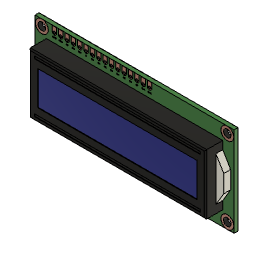
Control Panel v4 (Autodesk Fusion 360 archive; units mm, degrees)
design "LCD screen"
Autodesk Fusion 360 part; units mm, degrees
(part 1 of 2)
sketch "Boceto1" plane through (0, 0, 0) normal (0, 1, 0) x (1, 0, 0)
  line L0 (40.08, -18.04) -> (-40.08, -18.04)
  line L1 (-40.08, -18.04) -> (-40.08, 18.04)
  line L2 (-40.08, 18.04) -> (40.08, 18.04)
  line L3 (40.08, 18.04) -> (40.08, -18.04)
  line L4 (40.08, -18.04) -> (-40.08, 18.04) construction
  line L5 (-40.08, -18.04) -> (40.08, 18.04) construction
  dimension "d1" = 80.16
  dimension "d2" = 36.08
  constraint horizontal L0
  constraint perpendicular L0 L1
  constraint parallel L0 L2
  constraint parallel L1 L3
  constraint coincident L4 origin
  constraint coincident L5 origin
  measures "d1" distance of L0.start L0.end
  measures "d2" distance of L0.start L2.end
extrude "Extruir1" add sketch "Boceto1" along normal blind 1.61
sketch "Boceto2" plane through (0, 0, 0) normal (0, -1, 0) x (1, 0, 0)
  line L0 (-40.08, -18.04) -> (40.08, -18.04)
  line L1 (40.08, -18.04) -> (40.08, 18.04)
  line L2 (40.08, 18.04) -> (-40.08, 18.04)
  line L3 (-40.08, 18.04) -> (-40.08, -18.04)
  line L4 (0, 0) -> (0, 18.04) construction
  line L5 (0, 0) -> (40.08, 0) construction
  circle A0 centre (37.355, 15.465) radius 1.525
  circle A1 centre (37.355, 15.465) radius 2.595
  circle A2 centre (-37.355, 15.465) radius 1.525
  circle A3 centre (-37.355, 15.465) radius 2.595
  circle A4 centre (-37.355, -15.465) radius 1.525
  circle A5 centre (-37.355, -15.465) radius 2.595
  circle A6 centre (37.355, -15.465) radius 1.525
  circle A7 centre (37.355, -15.465) radius 2.595
  line L6 (35.525, 12.1) -> (-35.525, 12.1)
  line L7 (-35.525, 12.1) -> (-35.525, -12.1)
  line L8 (-35.525, -12.1) -> (35.525, -12.1)
  line L9 (35.525, -12.1) -> (35.525, 12.1)
  line L10 (35.525, 12.1) -> (-35.525, -12.1) construction
  line L11 (-35.525, 12.1) -> (35.525, -12.1) construction
  line L12 (35.525, 8.88) -> (38.695, 8.88)
  line L13 (38.695, 8.88) -> (38.695, -8.88)
  line L14 (38.695, -8.88) -> (35.525, -8.88)
  line L15 (35.525, -8.88) -> (35.525, 8.88)
  line L16 (38.695, 3.54) -> (35.525, 8.88)
  line L17 (38.695, -3.54) -> (35.525, -8.88)
  line L18 (-33.18, 17.94) -> (-31.43, 17.94)
  line L19 (-31.43, 17.94) -> (-31.43, 15.815)
  line L20 (-33.18, 15.815) -> (-33.18, 17.94)
  line L21 (-31.43, 17.94) -> (-33.18, 15.815) construction
  line L22 (-31.43, 15.815) -> (-33.18, 17.94) construction
  line L23 (-32.305, 14.94) -> (-33.18, 14.94) construction
  line L24 (-33.18, 15.815) -> (-33.18, 14.94) construction
  arc A8 (-33.18, 15.815) -> (-31.43, 15.815) centre (-32.305, 15.815) ccw
  line L25 (-32.305, 16.8775) -> (-32.305, 14.94) construction
  line L26 (-30.6233, 17.94) -> (-28.8733, 17.94)
  line L27 (-30.6233, 15.815) -> (-30.6233, 17.94)
  arc A9 (-30.6233, 15.815) -> (-28.8733, 15.815) centre (-29.7483, 15.815) ccw
  line L28 (-28.8733, 17.94) -> (-28.8733, 15.815)
  line L29 (-28.0667, 17.94) -> (-26.3167, 17.94)
  line L30 (-28.0667, 15.815) -> (-28.0667, 17.94)
  arc A10 (-28.0667, 15.815) -> (-26.3167, 15.815) centre (-27.1917, 15.815) ccw
  line L31 (-26.3167, 17.94) -> (-26.3167, 15.815)
  line L32 (-25.51, 17.94) -> (-23.76, 17.94)
  line L33 (-25.51, 15.815) -> (-25.51, 17.94)
  arc A11 (-25.51, 15.815) -> (-23.76, 15.815) centre (-24.635, 15.815) ccw
  line L34 (-23.76, 17.94) -> (-23.76, 15.815)
  line L35 (-22.9533, 17.94) -> (-21.2033, 17.94)
  line L36 (-22.9533, 15.815) -> (-22.9533, 17.94)
  arc A12 (-22.9533, 15.815) -> (-21.2033, 15.815) centre (-22.0783, 15.815) ccw
  line L37 (-21.2033, 17.94) -> (-21.2033, 15.815)
  line L38 (-20.3967, 17.94) -> (-18.6467, 17.94)
  line L39 (-20.3967, 15.815) -> (-20.3967, 17.94)
  arc A13 (-20.3967, 15.815) -> (-18.6467, 15.815) centre (-19.5217, 15.815) ccw
  line L40 (-18.6467, 17.94) -> (-18.6467, 15.815)
  line L41 (-17.84, 17.94) -> (-16.09, 17.94)
  line L42 (-17.84, 15.815) -> (-17.84, 17.94)
  arc A14 (-17.84, 15.815) -> (-16.09, 15.815) centre (-16.965, 15.815) ccw
  line L43 (-16.09, 17.94) -> (-16.09, 15.815)
  line L44 (-15.2833, 17.94) -> (-13.5333, 17.94)
  line L45 (-15.2833, 15.815) -> (-15.2833, 17.94)
  arc A15 (-15.2833, 15.815) -> (-13.5333, 15.815) centre (-14.4083, 15.815) ccw
  line L46 (-13.5333, 17.94) -> (-13.5333, 15.815)
  line L47 (-12.7267, 17.94) -> (-10.9767, 17.94)
  line L48 (-12.7267, 15.815) -> (-12.7267, 17.94)
  arc A16 (-12.7267, 15.815) -> (-10.9767, 15.815) centre (-11.8517, 15.815) ccw
  line L49 (-10.9767, 17.94) -> (-10.9767, 15.815)
  line L50 (-10.17, 17.94) -> (-8.42, 17.94)
  line L51 (-10.17, 15.815) -> (-10.17, 17.94)
  arc A17 (-10.17, 15.815) -> (-8.42, 15.815) centre (-9.295, 15.815) ccw
  line L52 (-8.42, 17.94) -> (-8.42, 15.815)
  line L53 (-7.6133, 17.94) -> (-5.8633, 17.94)
  line L54 (-7.6133, 15.815) -> (-7.6133, 17.94)
  arc A18 (-7.6133, 15.815) -> (-5.8633, 15.815) centre (-6.7383, 15.815) ccw
  line L55 (-5.8633, 17.94) -> (-5.8633, 15.815)
  line L56 (-5.0567, 17.94) -> (-3.3067, 17.94)
  line L57 (-5.0567, 15.815) -> (-5.0567, 17.94)
  arc A19 (-5.0567, 15.815) -> (-3.3067, 15.815) centre (-4.1817, 15.815) ccw
  line L58 (-3.3067, 17.94) -> (-3.3067, 15.815)
  line L59 (-2.5, 17.94) -> (-0.75, 17.94)
  line L60 (-2.5, 15.815) -> (-2.5, 17.94)
  arc A20 (-2.5, 15.815) -> (-0.75, 15.815) centre (-1.625, 15.815) ccw
  line L61 (-0.75, 17.94) -> (-0.75, 15.815)
  line L62 (0.0567, 17.94) -> (1.8067, 17.94)
  line L63 (0.0567, 15.815) -> (0.0567, 17.94)
  arc A21 (0.0567, 15.815) -> (1.8067, 15.815) centre (0.9317, 15.815) ccw
  line L64 (1.8067, 17.94) -> (1.8067, 15.815)
  line L65 (2.6133, 17.94) -> (4.3633, 17.94)
  line L66 (2.6133, 15.815) -> (2.6133, 17.94)
  arc A22 (2.6133, 15.815) -> (4.3633, 15.815) centre (3.4883, 15.815) ccw
  line L67 (4.3633, 17.94) -> (4.3633, 15.815)
  line L68 (5.17, 17.94) -> (6.92, 17.94)
  line L69 (5.17, 15.815) -> (5.17, 17.94)
  arc A23 (5.17, 15.815) -> (6.92, 15.815) centre (6.045, 15.815) ccw
  line L70 (6.92, 17.94) -> (6.92, 15.815)
  circle A24 centre (-32.305, 15.815) radius 0.5
  circle A25 centre (-29.7483, 15.815) radius 0.5
  circle A26 centre (-27.1917, 15.815) radius 0.5
  circle A27 centre (-24.635, 15.815) radius 0.5
  circle A28 centre (-22.0783, 15.815) radius 0.5
  circle A29 centre (-19.5217, 15.815) radius 0.5
  circle A30 centre (-16.965, 15.815) radius 0.5
  circle A31 centre (-14.4083, 15.815) radius 0.5
  circle A32 centre (-11.8517, 15.815) radius 0.5
  circle A33 centre (-9.295, 15.815) radius 0.5
  circle A34 centre (-6.7383, 15.815) radius 0.5
  circle A35 centre (-4.1817, 15.815) radius 0.5
  circle A36 centre (-1.625, 15.815) radius 0.5
  circle A37 centre (0.9317, 15.815) radius 0.5
  circle A38 centre (3.4883, 15.815) radius 0.5
  circle A39 centre (6.045, 15.815) radius 0.5
  line L71 (-32.305, 14.94) -> (-32.305, 12.1) construction
  line L72 (-33.18, 14.5) -> (-31.43, 14.5)
  line L73 (-31.43, 14.5) -> (-31.43, 13.6)
  line L74 (-31.43, 13.6) -> (-33.18, 13.6)
  line L75 (-33.18, 13.6) -> (-33.18, 14.5)
  line L76 (-30.6233, 14.5) -> (-28.8733, 14.5)
  line L77 (-30.6233, 13.6) -> (-30.6233, 14.5)
  line L78 (-28.8733, 13.6) -> (-30.6233, 13.6)
  line L79 (-28.8733, 14.5) -> (-28.8733, 13.6)
  line L80 (-28.0667, 14.5) -> (-26.3167, 14.5)
  line L81 (-28.0667, 13.6) -> (-28.0667, 14.5)
  line L82 (-26.3167, 13.6) -> (-28.0667, 13.6)
  line L83 (-26.3167, 14.5) -> (-26.3167, 13.6)
  line L84 (-25.51, 14.5) -> (-23.76, 14.5)
  line L85 (-25.51, 13.6) -> (-25.51, 14.5)
  line L86 (-23.76, 13.6) -> (-25.51, 13.6)
  line L87 (-23.76, 14.5) -> (-23.76, 13.6)
  line L88 (-22.9533, 14.5) -> (-21.2033, 14.5)
  line L89 (-22.9533, 13.6) -> (-22.9533, 14.5)
  line L90 (-21.2033, 13.6) -> (-22.9533, 13.6)
  line L91 (-21.2033, 14.5) -> (-21.2033, 13.6)
  line L92 (-20.3967, 14.5) -> (-18.6467, 14.5)
  line L93 (-20.3967, 13.6) -> (-20.3967, 14.5)
  line L94 (-18.6467, 13.6) -> (-20.3967, 13.6)
  line L95 (-18.6467, 14.5) -> (-18.6467, 13.6)
  line L96 (-17.84, 14.5) -> (-16.09, 14.5)
  line L97 (-17.84, 13.6) -> (-17.84, 14.5)
  line L98 (-16.09, 13.6) -> (-17.84, 13.6)
  line L99 (-16.09, 14.5) -> (-16.09, 13.6)
  line L100 (-15.2833, 14.5) -> (-13.5333, 14.5)
  line L101 (-15.2833, 13.6) -> (-15.2833, 14.5)
  line L102 (-13.5333, 13.6) -> (-15.2833, 13.6)
  line L103 (-13.5333, 14.5) -> (-13.5333, 13.6)
  line L104 (-12.7267, 14.5) -> (-10.9767, 14.5)
  line L105 (-12.7267, 13.6) -> (-12.7267, 14.5)
  line L106 (-10.9767, 13.6) -> (-12.7267, 13.6)
  line L107 (-10.9767, 14.5) -> (-10.9767, 13.6)
  line L108 (-10.17, 14.5) -> (-8.42, 14.5)
  line L109 (-10.17, 13.6) -> (-10.17, 14.5)
  line L110 (-8.42, 13.6) -> (-10.17, 13.6)
  line L111 (-8.42, 14.5) -> (-8.42, 13.6)
  line L112 (-7.6133, 14.5) -> (-5.8633, 14.5)
  line L113 (-7.6133, 13.6) -> (-7.6133, 14.5)
  line L114 (-5.8633, 13.6) -> (-7.6133, 13.6)
  line L115 (-5.8633, 14.5) -> (-5.8633, 13.6)
  line L116 (-5.0567, 14.5) -> (-3.3067, 14.5)
  line L117 (-5.0567, 13.6) -> (-5.0567, 14.5)
  line L118 (-3.3067, 13.6) -> (-5.0567, 13.6)
  line L119 (-3.3067, 14.5) -> (-3.3067, 13.6)
  line L120 (-2.5, 14.5) -> (-0.75, 14.5)
  line L121 (-2.5, 13.6) -> (-2.5, 14.5)
  line L122 (-0.75, 13.6) -> (-2.5, 13.6)
  line L123 (-0.75, 14.5) -> (-0.75, 13.6)
  line L124 (0.0567, 14.5) -> (1.8067, 14.5)
  line L125 (0.0567, 13.6) -> (0.0567, 14.5)
  line L126 (1.8067, 13.6) -> (0.0567, 13.6)
  line L127 (1.8067, 14.5) -> (1.8067, 13.6)
  line L128 (2.6133, 14.5) -> (4.3633, 14.5)
  line L129 (2.6133, 13.6) -> (2.6133, 14.5)
  line L130 (4.3633, 13.6) -> (2.6133, 13.6)
  line L131 (4.3633, 14.5) -> (4.3633, 13.6)
  line L132 (5.17, 14.5) -> (6.92, 14.5)
  line L133 (5.17, 13.6) -> (5.17, 14.5)
  line L134 (6.92, 13.6) -> (5.17, 13.6)
  line L135 (6.92, 14.5) -> (6.92, 13.6)
  line L136 (-32.7932, 13.9961) -> (-32.7932, 14.0548)
  line L137 (-32.7932, 14.0548) -> (-32.5814, 14.0551)
  line L138 (-32.5814, 14.0551) -> (-32.5814, 13.8696)
  spline S0 degree 2 poles (-32.5814, 13.8696) (-32.6302, 13.8307) (-32.682, 13.8111) knots 0 0 0 1 1 1
  spline S1 degree 2 poles (-32.682, 13.8111) (-32.7339, 13.7915) (-32.7885, 13.7915) knots 0 0 0 1 1 1
  spline S2 degree 2 poles (-32.7885, 13.7915) (-32.8621, 13.7915) (-32.9223, 13.823) knots 0 0 0 1 1 1
  spline S3 degree 2 poles (-32.9223, 13.823) (-32.9825, 13.8546) (-33.0132, 13.9143) knots 0 0 0 1 1 1
  spline S4 degree 2 poles (-33.0132, 13.9143) (-33.0439, 13.9739) (-33.0439, 14.0476) knots 0 0 0 1 1 1
  spline S5 degree 2 poles (-33.0439, 14.0476) (-33.0439, 14.1206) (-33.0134, 14.1839) knots 0 0 0 1 1 1
  spline S6 degree 2 poles (-33.0134, 14.1839) (-32.9829, 14.2471) (-32.9256, 14.2778) knots 0 0 0 1 1 1
  spline S7 degree 2 poles (-32.9256, 14.2778) (-32.8683, 14.3085) (-32.7936, 14.3085) knots 0 0 0 1 1 1
  spline S8 degree 2 poles (-32.7936, 14.3085) (-32.7393, 14.3085) (-32.6955, 14.291) knots 0 0 0 1 1 1
  spline S9 degree 2 poles (-32.6955, 14.291) (-32.6517, 14.2734) (-32.6268, 14.242) knots 0 0 0 1 1 1
  spline S10 degree 2 poles (-32.6268, 14.242) (-32.6019, 14.2106) (-32.5889, 14.1602) knots 0 0 0 1 1 1
  line L139 (-32.5889, 14.1602) -> (-32.6486, 14.1438)
  spline S11 degree 2 poles (-32.6486, 14.1438) (-32.6599, 14.182) (-32.6766, 14.2038) knots 0 0 0 1 1 1
  spline S12 degree 2 poles (-32.6766, 14.2038) (-32.6933, 14.2256) (-32.7243, 14.2388) knots 0 0 0 1 1 1
  spline S13 degree 2 poles (-32.7243, 14.2388) (-32.7554, 14.2519) (-32.7932, 14.2519) knots 0 0 0 1 1 1
  spline S14 degree 2 poles (-32.7932, 14.2519) (-32.8386, 14.2519) (-32.8717, 14.2381) knots 0 0 0 1 1 1
  spline S15 degree 2 poles (-32.8717, 14.2381) (-32.9048, 14.2243) (-32.9251, 14.2018) knots 0 0 0 1 1 1
  spline S16 degree 2 poles (-32.9251, 14.2018) (-32.9453, 14.1793) (-32.9566, 14.1523) knots 0 0 0 1 1 1
  spline S17 degree 2 poles (-32.9566, 14.1523) (-32.9757, 14.1059) (-32.9757, 14.0517) knots 0 0 0 1 1 1
  spline S18 degree 2 poles (-32.9757, 14.0517) (-32.9757, 13.9849) (-32.9527, 13.9398) knots 0 0 0 1 1 1
  spline S19 degree 2 poles (-32.9527, 13.9398) (-32.9297, 13.8948) (-32.8857, 13.873) knots 0 0 0 1 1 1
  spline S20 degree 2 poles (-32.8857, 13.873) (-32.8417, 13.8512) (-32.7922, 13.8512) knots 0 0 0 1 1 1
  spline S21 degree 2 poles (-32.7922, 13.8512) (-32.7492, 13.8512) (-32.7083, 13.8677) knots 0 0 0 1 1 1
  spline S22 degree 2 poles (-32.7083, 13.8677) (-32.6674, 13.8842) (-32.6462, 13.903) knots 0 0 0 1 1 1
  line L140 (-32.6462, 13.903) -> (-32.6462, 13.9961)
  line L141 (-32.6462, 13.9961) -> (-32.7932, 13.9961)
  line L142 (-32.4846, 13.8) -> (-32.4846, 14.3)
  line L143 (-32.4846, 14.3) -> (-32.4167, 14.3)
  line L144 (-32.4167, 14.3) -> (-32.1541, 13.9074)
  line L145 (-32.1541, 13.9074) -> (-32.1541, 14.3)
  line L146 (-32.1541, 14.3) -> (-32.0906, 14.3)
  line L147 (-32.0906, 14.3) -> (-32.0906, 13.8)
  line L148 (-32.0906, 13.8) -> (-32.1585, 13.8)
  line L149 (-32.1585, 13.8) -> (-32.4211, 14.1929)
  line L150 (-32.4211, 14.1929) -> (-32.4211, 13.8)
  line L151 (-32.4211, 13.8) -> (-32.4846, 13.8)
  line L152 (-31.9795, 13.8) -> (-31.9795, 14.3)
  line L153 (-31.9795, 14.3) -> (-31.8072, 14.3)
  spline S23 degree 2 poles (-31.8072, 14.3) (-31.7489, 14.3) (-31.7182, 14.2928) knots 0 0 0 1 1 1
  spline S24 degree 2 poles (-31.7182, 14.2928) (-31.6752, 14.2829) (-31.6449, 14.257) knots 0 0 0 1 1 1
  spline S25 degree 2 poles (-31.6449, 14.257) (-31.6053, 14.2236) (-31.5857, 14.1716) knots 0 0 0 1 1 1
  spline S26 degree 2 poles (-31.5857, 14.1716) (-31.5661, 14.1196) (-31.5661, 14.0527) knots 0 0 0 1 1 1
  spline S27 degree 2 poles (-31.5661, 14.0527) (-31.5661, 13.9958) (-31.5794, 13.9518) knots 0 0 0 1 1 1
  spline S28 degree 2 poles (-31.5794, 13.9518) (-31.5927, 13.9078) (-31.6135, 13.879) knots 0 0 0 1 1 1
  spline S29 degree 2 poles (-31.6135, 13.879) (-31.6343, 13.8501) (-31.659, 13.8336) knots 0 0 0 1 1 1
  spline S30 degree 2 poles (-31.659, 13.8336) (-31.6838, 13.8171) (-31.7187, 13.8085) knots 0 0 0 1 1 1
  spline S31 degree 2 poles (-31.7187, 13.8085) (-31.7537, 13.8) (-31.799, 13.8) knots 0 0 0 1 1 1
  line L154 (-31.799, 13.8) -> (-31.9795, 13.8)
  line L155 (-31.9133, 13.859) -> (-31.8065, 13.859)
  spline S32 degree 2 poles (-31.8065, 13.859) (-31.7571, 13.859) (-31.7289, 13.8682) knots 0 0 0 1 1 1
  spline S33 degree 2 poles (-31.7289, 13.8682) (-31.7008, 13.8774) (-31.6841, 13.8941) knots 0 0 0 1 1 1
  spline S34 degree 2 poles (-31.6841, 13.8941) (-31.6606, 13.9177) (-31.6474, 13.9574) knots 0 0 0 1 1 1
  spline S35 degree 2 poles (-31.6474, 13.9574) (-31.6343, 13.9971) (-31.6343, 14.0538) knots 0 0 0 1 1 1
  spline S36 degree 2 poles (-31.6343, 14.0538) (-31.6343, 14.1322) (-31.66, 14.1743) knots 0 0 0 1 1 1
  spline S37 degree 2 poles (-31.66, 14.1743) (-31.6858, 14.2164) (-31.7226, 14.2308) knots 0 0 0 1 1 1
  spline S38 degree 2 poles (-31.7226, 14.2308) (-31.7492, 14.241) (-31.8082, 14.241) knots 0 0 0 1 1 1
  line L156 (-31.8082, 14.241) -> (-31.9133, 14.241)
  line L157 (-31.9133, 14.241) -> (-31.9133, 13.859)
  line L158 (-30.2719, 13.8) -> (-30.4656, 14.3)
  line L159 (-30.4656, 14.3) -> (-30.394, 14.3)
  line L160 (-30.394, 14.3) -> (-30.264, 13.9368)
  spline S39 degree 2 poles (-30.264, 13.9368) (-30.2483, 13.8931) (-30.2378, 13.8549) knots 0 0 0 1 1 1
  spline S40 degree 2 poles (-30.2378, 13.8549) (-30.2262, 13.8958) (-30.2108, 13.9368) knots 0 0 0 1 1 1
  line L161 (-30.2108, 13.9368) -> (-30.0758, 14.3)
  line L162 (-30.0758, 14.3) -> (-30.0082, 14.3)
  line L163 (-30.0082, 14.3) -> (-30.204, 13.8)
  line L164 (-30.204, 13.8) -> (-30.2719, 13.8)
  line L165 (-29.9489, 13.8) -> (-29.9489, 14.3)
  line L166 (-29.9489, 14.3) -> (-29.7766, 14.3)
  spline S41 degree 2 poles (-29.7766, 14.3) (-29.7183, 14.3) (-29.6876, 14.2928) knots 0 0 0 1 1 1
  spline S42 degree 2 poles (-29.6876, 14.2928) (-29.6446, 14.2829) (-29.6143, 14.257) knots 0 0 0 1 1 1
  spline S43 degree 2 poles (-29.6143, 14.257) (-29.5747, 14.2236) (-29.5551, 14.1716) knots 0 0 0 1 1 1
  spline S44 degree 2 poles (-29.5551, 14.1716) (-29.5355, 14.1196) (-29.5355, 14.0527) knots 0 0 0 1 1 1
  spline S45 degree 2 poles (-29.5355, 14.0527) (-29.5355, 13.9958) (-29.5488, 13.9518) knots 0 0 0 1 1 1
  spline S46 degree 2 poles (-29.5488, 13.9518) (-29.5621, 13.9078) (-29.5829, 13.879) knots 0 0 0 1 1 1
  spline S47 degree 2 poles (-29.5829, 13.879) (-29.6037, 13.8501) (-29.6284, 13.8336) knots 0 0 0 1 1 1
  spline S48 degree 2 poles (-29.6284, 13.8336) (-29.6532, 13.8171) (-29.6881, 13.8085) knots 0 0 0 1 1 1
  spline S49 degree 2 poles (-29.6881, 13.8085) (-29.7231, 13.8) (-29.7685, 13.8) knots 0 0 0 1 1 1
  line L167 (-29.7685, 13.8) -> (-29.9489, 13.8)
  line L168 (-29.8827, 13.859) -> (-29.776, 13.859)
  spline S50 degree 2 poles (-29.776, 13.859) (-29.7265, 13.859) (-29.6984, 13.8682) knots 0 0 0 1 1 1
  spline S51 degree 2 poles (-29.6984, 13.8682) (-29.6702, 13.8774) (-29.6535, 13.8941) knots 0 0 0 1 1 1
  spline S52 degree 2 poles (-29.6535, 13.8941) (-29.63, 13.9177) (-29.6169, 13.9574) knots 0 0 0 1 1 1
  spline S53 degree 2 poles (-29.6169, 13.9574) (-29.6037, 13.9971) (-29.6037, 14.0538) knots 0 0 0 1 1 1
  spline S54 degree 2 poles (-29.6037, 14.0538) (-29.6037, 14.1322) (-29.6295, 14.1743) knots 0 0 0 1 1 1
  spline S55 degree 2 poles (-29.6295, 14.1743) (-29.6552, 14.2164) (-29.6921, 14.2308) knots 0 0 0 1 1 1
  spline S56 degree 2 poles (-29.6921, 14.2308) (-29.7187, 14.241) (-29.7777, 14.241) knots 0 0 0 1 1 1
  line L169 (-29.7777, 14.241) -> (-29.8827, 14.241)
  line L170 (-29.8827, 14.241) -> (-29.8827, 13.859)
  line L171 (-29.4444, 13.8) -> (-29.4444, 14.3)
  line L172 (-29.4444, 14.3) -> (-29.2722, 14.3)
  spline S57 degree 2 poles (-29.2722, 14.3) (-29.2139, 14.3) (-29.1832, 14.2928) knots 0 0 0 1 1 1
  spline S58 degree 2 poles (-29.1832, 14.2928) (-29.1402, 14.2829) (-29.1099, 14.257) knots 0 0 0 1 1 1
  spline S59 degree 2 poles (-29.1099, 14.257) (-29.0703, 14.2236) (-29.0507, 14.1716) knots 0 0 0 1 1 1
  spline S60 degree 2 poles (-29.0507, 14.1716) (-29.0311, 14.1196) (-29.0311, 14.0527) knots 0 0 0 1 1 1
  spline S61 degree 2 poles (-29.0311, 14.0527) (-29.0311, 13.9958) (-29.0444, 13.9518) knots 0 0 0 1 1 1
  spline S62 degree 2 poles (-29.0444, 13.9518) (-29.0577, 13.9078) (-29.0785, 13.879) knots 0 0 0 1 1 1
  spline S63 degree 2 poles (-29.0785, 13.879) (-29.0993, 13.8501) (-29.124, 13.8336) knots 0 0 0 1 1 1
  spline S64 degree 2 poles (-29.124, 13.8336) (-29.1487, 13.8171) (-29.1837, 13.8085) knots 0 0 0 1 1 1
  spline S65 degree 2 poles (-29.1837, 13.8085) (-29.2187, 13.8) (-29.264, 13.8) knots 0 0 0 1 1 1
  line L173 (-29.264, 13.8) -> (-29.4444, 13.8)
  line L174 (-29.3783, 13.859) -> (-29.2715, 13.859)
  spline S66 degree 2 poles (-29.2715, 13.859) (-29.2221, 13.859) (-29.1939, 13.8682) knots 0 0 0 1 1 1
  spline S67 degree 2 poles (-29.1939, 13.8682) (-29.1658, 13.8774) (-29.1491, 13.8941) knots 0 0 0 1 1 1
  spline S68 degree 2 poles (-29.1491, 13.8941) (-29.1256, 13.9177) (-29.1124, 13.9574) knots 0 0 0 1 1 1
  spline S69 degree 2 poles (-29.1124, 13.9574) (-29.0993, 13.9971) (-29.0993, 14.0538) knots 0 0 0 1 1 1
  spline S70 degree 2 poles (-29.0993, 14.0538) (-29.0993, 14.1322) (-29.125, 14.1743) knots 0 0 0 1 1 1
  spline S71 degree 2 poles (-29.125, 14.1743) (-29.1508, 14.2164) (-29.1876, 14.2308) knots 0 0 0 1 1 1
  spline S72 degree 2 poles (-29.1876, 14.2308) (-29.2142, 14.241) (-29.2732, 14.241) knots 0 0 0 1 1 1
  line L175 (-29.2732, 14.241) -> (-29.3783, 14.241)
  line L176 (-29.3783, 14.241) -> (-29.3783, 13.859)
  line L177 (-27.4069, 13.8) -> (-27.6006, 14.3)
  line L178 (-27.6006, 14.3) -> (-27.529, 14.3)
  line L179 (-27.529, 14.3) -> (-27.399, 13.9368)
  spline S73 degree 2 poles (-27.399, 13.9368) (-27.3833, 13.8931) (-27.3728, 13.8549) knots 0 0 0 1 1 1
  spline S74 degree 2 poles (-27.3728, 13.8549) (-27.3612, 13.8958) (-27.3458, 13.9368) knots 0 0 0 1 1 1
  line L180 (-27.3458, 13.9368) -> (-27.2108, 14.3)
  line L181 (-27.2108, 14.3) -> (-27.1432, 14.3)
  line L182 (-27.1432, 14.3) -> (-27.339, 13.8)
  line L183 (-27.339, 13.8) -> (-27.4069, 13.8)
  spline S75 degree 2 poles (-27.1088, 14.0466) (-27.1088, 14.1353) (-27.0905, 14.1893) knots 0 0 0 1 1 1
  spline S76 degree 2 poles (-27.0905, 14.1893) (-27.0723, 14.2434) (-27.0363, 14.2727) knots 0 0 0 1 1 1
  spline S77 degree 2 poles (-27.0363, 14.2727) (-27.0003, 14.302) (-26.9458, 14.302) knots 0 0 0 1 1 1
  spline S78 degree 2 poles (-26.9458, 14.302) (-26.9055, 14.302) (-26.8752, 14.2858) knots 0 0 0 1 1 1
  spline S79 degree 2 poles (-26.8752, 14.2858) (-26.8448, 14.2696) (-26.825, 14.2391) knots 0 0 0 1 1 1
  spline S80 degree 2 poles (-26.825, 14.2391) (-26.8052, 14.2086) (-26.794, 14.1648) knots 0 0 0 1 1 1
  spline S81 degree 2 poles (-26.794, 14.1648) (-26.7827, 14.1209) (-26.7827, 14.0466) knots 0 0 0 1 1 1
  spline S82 degree 2 poles (-26.7827, 14.0466) (-26.7827, 13.9586) (-26.8008, 13.9045) knots 0 0 0 1 1 1
  spline S83 degree 2 poles (-26.8008, 13.9045) (-26.8189, 13.8505) (-26.8549, 13.821) knots 0 0 0 1 1 1
  spline S84 degree 2 poles (-26.8549, 13.821) (-26.8908, 13.7915) (-26.9458, 13.7915) knots 0 0 0 1 1 1
  spline S85 degree 2 poles (-26.9458, 13.7915) (-27.0181, 13.7915) (-27.0593, 13.8433) knots 0 0 0 1 1 1
  spline S86 degree 2 poles (-27.0593, 13.8433) (-27.1088, 13.9057) (-27.1088, 14.0466) knots 0 0 0 1 1 1
  spline S87 degree 2 poles (-27.0457, 14.0466) (-27.0457, 13.9235) (-27.0169, 13.8827) knots 0 0 0 1 1 1
  spline S88 degree 2 poles (-27.0169, 13.8827) (-26.9881, 13.842) (-26.9458, 13.842) knots 0 0 0 1 1 1
  spline S89 degree 2 poles (-26.9458, 13.842) (-26.9035, 13.842) (-26.8746, 13.8829) knots 0 0 0 1 1 1
  spline S90 degree 2 poles (-26.8746, 13.8829) (-26.8458, 13.9238) (-26.8458, 14.0466) knots 0 0 0 1 1 1
  spline S91 degree 2 poles (-26.8458, 14.0466) (-26.8458, 14.1701) (-26.8746, 14.2106) knots 0 0 0 1 1 1
  spline S92 degree 2 poles (-26.8746, 14.2106) (-26.9035, 14.2512) (-26.9464, 14.2512) knots 0 0 0 1 1 1
  spline S93 degree 2 poles (-26.9464, 14.2512) (-26.9887, 14.2512) (-27.014, 14.2154) knots 0 0 0 1 1 1
  spline S94 degree 2 poles (-27.014, 14.2154) (-27.0457, 14.1697) (-27.0457, 14.0466) knots 0 0 0 1 1 1
  line L184 (-25.0745, 13.8) -> (-25.0745, 14.3)
  line L185 (-25.0745, 14.3) -> (-24.8528, 14.3)
  spline S95 degree 2 poles (-24.8528, 14.3) (-24.7859, 14.3) (-24.7511, 14.2865) knots 0 0 0 1 1 1
  spline S96 degree 2 poles (-24.7511, 14.2865) (-24.7163, 14.2731) (-24.6955, 14.2389) knots 0 0 0 1 1 1
  spline S97 degree 2 poles (-24.6955, 14.2389) (-24.6747, 14.2048) (-24.6747, 14.1636) knots 0 0 0 1 1 1
  spline S98 degree 2 poles (-24.6747, 14.1636) (-24.6747, 14.1104) (-24.7092, 14.0739) knots 0 0 0 1 1 1
  spline S99 degree 2 poles (-24.7092, 14.0739) (-24.7436, 14.0374) (-24.8156, 14.0275) knots 0 0 0 1 1 1
  spline S100 degree 2 poles (-24.8156, 14.0275) (-24.7893, 14.0149) (-24.7757, 14.0026) knots 0 0 0 1 1 1
  spline S101 degree 2 poles (-24.7757, 14.0026) (-24.7467, 13.976) (-24.7208, 13.9361) knots 0 0 0 1 1 1
  line L186 (-24.7208, 13.9361) -> (-24.6338, 13.8)
  line L187 (-24.6338, 13.8) -> (-24.717, 13.8)
  line L188 (-24.717, 13.8) -> (-24.7832, 13.904)
  spline S102 degree 2 poles (-24.7832, 13.904) (-24.8122, 13.949) (-24.8309, 13.9729) knots 0 0 0 1 1 1
  spline S103 degree 2 poles (-24.8309, 13.9729) (-24.8497, 13.9968) (-24.8645, 14.0063) knots 0 0 0 1 1 1
  spline S104 degree 2 poles (-24.8645, 14.0063) (-24.8794, 14.0159) (-24.8947, 14.0196) knots 0 0 0 1 1 1
  spline S105 degree 2 poles (-24.8947, 14.0196) (-24.906, 14.022) (-24.9316, 14.022) knots 0 0 0 1 1 1
  line L189 (-24.9316, 14.022) -> (-25.0083, 14.022)
  line L190 (-25.0083, 14.022) -> (-25.0083, 13.8)
  line L191 (-25.0083, 13.8) -> (-25.0745, 13.8)
  line L192 (-25.0083, 14.0793) -> (-24.8661, 14.0793)
  spline S106 degree 2 poles (-24.8661, 14.0793) (-24.8207, 14.0793) (-24.7951, 14.0887) knots 0 0 0 1 1 1
  spline S107 degree 2 poles (-24.7951, 14.0887) (-24.7695, 14.0981) (-24.7562, 14.1187) knots 0 0 0 1 1 1
  spline S108 degree 2 poles (-24.7562, 14.1187) (-24.7429, 14.1394) (-24.7429, 14.1636) knots 0 0 0 1 1 1
  spline S109 degree 2 poles (-24.7429, 14.1636) (-24.7429, 14.199) (-24.7687, 14.2219) knots 0 0 0 1 1 1
  spline S110 degree 2 poles (-24.7687, 14.2219) (-24.7944, 14.2447) (-24.85, 14.2447) knots 0 0 0 1 1 1
  line L193 (-24.85, 14.2447) -> (-25.0083, 14.2447)
  line L194 (-25.0083, 14.2447) -> (-25.0083, 14.0793)
  line L195 (-24.5936, 13.9606) -> (-24.5311, 13.9661)
  spline S111 degree 2 poles (-24.5311, 13.9661) (-24.5267, 13.9286) (-24.5105, 13.9045) knots 0 0 0 1 1 1
  spline S112 degree 2 poles (-24.5105, 13.9045) (-24.4943, 13.8805) (-24.4602, 13.8657) knots 0 0 0 1 1 1
  spline S113 degree 2 poles (-24.4602, 13.8657) (-24.4261, 13.8508) (-24.3835, 13.8508) knots 0 0 0 1 1 1
  spline S114 degree 2 poles (-24.3835, 13.8508) (-24.3456, 13.8508) (-24.3166, 13.8621) knots 0 0 0 1 1 1
  spline S115 degree 2 poles (-24.3166, 13.8621) (-24.2876, 13.8733) (-24.2735, 13.8929) knots 0 0 0 1 1 1
  spline S116 degree 2 poles (-24.2735, 13.8929) (-24.2593, 13.9126) (-24.2593, 13.9357) knots 0 0 0 1 1 1
  spline S117 degree 2 poles (-24.2593, 13.9357) (-24.2593, 13.9593) (-24.273, 13.9768) knots 0 0 0 1 1 1
  spline S118 degree 2 poles (-24.273, 13.9768) (-24.2866, 13.9944) (-24.318, 14.0063) knots 0 0 0 1 1 1
  spline S119 degree 2 poles (-24.318, 14.0063) (-24.3381, 14.0142) (-24.407, 14.0307) knots 0 0 0 1 1 1
  spline S120 degree 2 poles (-24.407, 14.0307) (-24.4759, 14.0473) (-24.5035, 14.0619) knots 0 0 0 1 1 1
  spline S121 degree 2 poles (-24.5035, 14.0619) (-24.5393, 14.0807) (-24.5569, 14.1085) knots 0 0 0 1 1 1
  spline S122 degree 2 poles (-24.5569, 14.1085) (-24.5745, 14.1363) (-24.5745, 14.1707) knots 0 0 0 1 1 1
  spline S123 degree 2 poles (-24.5745, 14.1707) (-24.5745, 14.2086) (-24.553, 14.2415) knots 0 0 0 1 1 1
  spline S124 degree 2 poles (-24.553, 14.2415) (-24.5315, 14.2744) (-24.4902, 14.2915) knots 0 0 0 1 1 1
  spline S125 degree 2 poles (-24.4902, 14.2915) (-24.4489, 14.3085) (-24.3985, 14.3085) knots 0 0 0 1 1 1
  spline S126 degree 2 poles (-24.3985, 14.3085) (-24.3429, 14.3085) (-24.3004, 14.2906) knots 0 0 0 1 1 1
  spline S127 degree 2 poles (-24.3004, 14.2906) (-24.258, 14.2727) (-24.2351, 14.2379) knots 0 0 0 1 1 1
  spline S128 degree 2 poles (-24.2351, 14.2379) (-24.2123, 14.2031) (-24.2105, 14.1591) knots 0 0 0 1 1 1
  line L196 (-24.2105, 14.1591) -> (-24.274, 14.1544)
  spline S129 degree 2 poles (-24.274, 14.1544) (-24.2791, 14.2018) (-24.3086, 14.226) knots 0 0 0 1 1 1
  spline S130 degree 2 poles (-24.3086, 14.226) (-24.3381, 14.2502) (-24.3957, 14.2502) knots 0 0 0 1 1 1
  spline S131 degree 2 poles (-24.3957, 14.2502) (-24.4558, 14.2502) (-24.4832, 14.2282) knots 0 0 0 1 1 1
  spline S132 degree 2 poles (-24.4832, 14.2282) (-24.5107, 14.2062) (-24.5107, 14.1752) knots 0 0 0 1 1 1
  spline S133 degree 2 poles (-24.5107, 14.1752) (-24.5107, 14.1482) (-24.4912, 14.1308) knots 0 0 0 1 1 1
  spline S134 degree 2 poles (-24.4912, 14.1308) (-24.4721, 14.1134) (-24.3915, 14.0952) knots 0 0 0 1 1 1
  spline S135 degree 2 poles (-24.3915, 14.0952) (-24.3108, 14.0769) (-24.2808, 14.0633) knots 0 0 0 1 1 1
  spline S136 degree 2 poles (-24.2808, 14.0633) (-24.2371, 14.0432) (-24.2163, 14.0123) knots 0 0 0 1 1 1
  spline S137 degree 2 poles (-24.2163, 14.0123) (-24.1955, 13.9814) (-24.1955, 13.9412) knots 0 0 0 1 1 1
  spline S138 degree 2 poles (-24.1955, 13.9412) (-24.1955, 13.9013) (-24.2184, 13.866) knots 0 0 0 1 1 1
  spline S139 degree 2 poles (-24.2184, 13.866) (-24.2412, 13.8307) (-24.284, 13.8111) knots 0 0 0 1 1 1
  spline S140 degree 2 poles (-24.284, 13.8111) (-24.3268, 13.7915) (-24.3804, 13.7915) knots 0 0 0 1 1 1
  spline S141 degree 2 poles (-24.3804, 13.7915) (-24.4483, 13.7915) (-24.4941, 13.8113) knots 0 0 0 1 1 1
  spline S142 degree 2 poles (-24.4941, 13.8113) (-24.54, 13.831) (-24.5661, 13.8708) knots 0 0 0 1 1 1
  spline S143 degree 2 poles (-24.5661, 13.8708) (-24.5922, 13.9105) (-24.5936, 13.9606) knots 0 0 0 1 1 1
  line L197 (-22.6225, 13.8) -> (-22.6225, 14.3)
  line L198 (-22.6225, 14.3) -> (-22.4008, 14.3)
  spline S144 degree 2 poles (-22.4008, 14.3) (-22.334, 14.3) (-22.2992, 14.2865) knots 0 0 0 1 1 1
  spline S145 degree 2 poles (-22.2992, 14.2865) (-22.2644, 14.2731) (-22.2436, 14.2389) knots 0 0 0 1 1 1
  spline S146 degree 2 poles (-22.2436, 14.2389) (-22.2228, 14.2048) (-22.2228, 14.1636) knots 0 0 0 1 1 1
  spline S147 degree 2 poles (-22.2228, 14.1636) (-22.2228, 14.1104) (-22.2572, 14.0739) knots 0 0 0 1 1 1
  spline S148 degree 2 poles (-22.2572, 14.0739) (-22.2917, 14.0374) (-22.3636, 14.0275) knots 0 0 0 1 1 1
  spline S149 degree 2 poles (-22.3636, 14.0275) (-22.3374, 14.0149) (-22.3237, 14.0026) knots 0 0 0 1 1 1
  spline S150 degree 2 poles (-22.3237, 14.0026) (-22.2947, 13.976) (-22.2688, 13.9361) knots 0 0 0 1 1 1
  line L199 (-22.2688, 13.9361) -> (-22.1818, 13.8)
  line L200 (-22.1818, 13.8) -> (-22.2651, 13.8)
  line L201 (-22.2651, 13.8) -> (-22.3312, 13.904)
  spline S151 degree 2 poles (-22.3312, 13.904) (-22.3602, 13.949) (-22.379, 13.9729) knots 0 0 0 1 1 1
  spline S152 degree 2 poles (-22.379, 13.9729) (-22.3977, 13.9968) (-22.4126, 14.0063) knots 0 0 0 1 1 1
  spline S153 degree 2 poles (-22.4126, 14.0063) (-22.4274, 14.0159) (-22.4428, 14.0196) knots 0 0 0 1 1 1
  spline S154 degree 2 poles (-22.4428, 14.0196) (-22.454, 14.022) (-22.4796, 14.022) knots 0 0 0 1 1 1
  line L202 (-22.4796, 14.022) -> (-22.5563, 14.022)
  line L203 (-22.5563, 14.022) -> (-22.5563, 13.8)
  line L204 (-22.5563, 13.8) -> (-22.6225, 13.8)
  line L205 (-22.5563, 14.0793) -> (-22.4141, 14.0793)
  spline S155 degree 2 poles (-22.4141, 14.0793) (-22.3687, 14.0793) (-22.3432, 14.0887) knots 0 0 0 1 1 1
  spline S156 degree 2 poles (-22.3432, 14.0887) (-22.3176, 14.0981) (-22.3043, 14.1187) knots 0 0 0 1 1 1
  spline S157 degree 2 poles (-22.3043, 14.1187) (-22.291, 14.1394) (-22.291, 14.1636) knots 0 0 0 1 1 1
  spline S158 degree 2 poles (-22.291, 14.1636) (-22.291, 14.199) (-22.3167, 14.2219) knots 0 0 0 1 1 1
  spline S159 degree 2 poles (-22.3167, 14.2219) (-22.3425, 14.2447) (-22.3981, 14.2447) knots 0 0 0 1 1 1
  line L206 (-22.3981, 14.2447) -> (-22.5563, 14.2447)
  line L207 (-22.5563, 14.2447) -> (-22.5563, 14.0793)
  line L208 (-22.0444, 13.8) -> (-22.1771, 14.3)
  line L209 (-22.1771, 14.3) -> (-22.1092, 14.3)
  line L210 (-22.1092, 14.3) -> (-22.0331, 13.9722)
  spline S160 degree 2 poles (-22.0331, 13.9722) (-22.0209, 13.9207) (-22.012, 13.8699) knots 0 0 0 1 1 1
  spline S161 degree 2 poles (-22.012, 13.8699) (-21.9929, 13.9501) (-21.9895, 13.9623) knots 0 0 0 1 1 1
  line L211 (-21.9895, 13.9623) -> (-21.8943, 14.3)
  line L212 (-21.8943, 14.3) -> (-21.8145, 14.3)
  line L213 (-21.8145, 14.3) -> (-21.7429, 14.0469)
  spline S162 degree 2 poles (-21.7429, 14.0469) (-21.716, 13.9528) (-21.704, 13.8699) knots 0 0 0 1 1 1
  spline S163 degree 2 poles (-21.704, 13.8699) (-21.6945, 13.9173) (-21.6791, 13.9787) knots 0 0 0 1 1 1
  line L214 (-21.6791, 13.9787) -> (-21.6007, 14.3)
  line L215 (-21.6007, 14.3) -> (-21.5342, 14.3)
  line L216 (-21.5342, 14.3) -> (-21.6713, 13.8)
  line L217 (-21.6713, 13.8) -> (-21.7351, 13.8)
  line L218 (-21.7351, 13.8) -> (-21.8404, 14.181)
  spline S164 degree 2 poles (-21.8404, 14.181) (-21.8537, 14.2287) (-21.8561, 14.2396) knots 0 0 0 1 1 1
  spline S165 degree 2 poles (-21.8561, 14.2396) (-21.864, 14.2052) (-21.8708, 14.181) knots 0 0 0 1 1 1
  line L219 (-21.8708, 14.181) -> (-21.9769, 13.8)
  line L220 (-21.9769, 13.8) -> (-22.0444, 13.8)
  line L221 (-19.7082, 13.8) -> (-19.7082, 14.3)
  line L222 (-19.7082, 14.3) -> (-19.3467, 14.3)
  line L223 (-19.3467, 14.3) -> (-19.3467, 14.241)
  line L224 (-19.3467, 14.241) -> (-19.6421, 14.241)
  line L225 (-19.6421, 14.241) -> (-19.6421, 14.0879)
  line L226 (-19.6421, 14.0879) -> (-19.3655, 14.0879)
  line L227 (-19.3655, 14.0879) -> (-19.3655, 14.0292)
  line L228 (-19.3655, 14.0292) -> (-19.6421, 14.0292)
  line L229 (-19.6421, 14.0292) -> (-19.6421, 13.859)
  line L230 (-19.6421, 13.859) -> (-19.3351, 13.859)
  line L231 (-19.3351, 13.859) -> (-19.3351, 13.8)
  line L232 (-19.3351, 13.8) -> (-19.7082, 13.8)
  line L233 (-17.3678, 13.8) -> (-17.3678, 14.3)
  line L234 (-17.3678, 14.3) -> (-17.1956, 14.3)
  spline S166 degree 2 poles (-17.1956, 14.3) (-17.1372, 14.3) (-17.1065, 14.2928) knots 0 0 0 1 1 1
  spline S167 degree 2 poles (-17.1065, 14.2928) (-17.0636, 14.2829) (-17.0332, 14.257) knots 0 0 0 1 1 1
  spline S168 degree 2 poles (-17.0332, 14.257) (-16.9936, 14.2236) (-16.974, 14.1716) knots 0 0 0 1 1 1
  spline S169 degree 2 poles (-16.974, 14.1716) (-16.9544, 14.1196) (-16.9544, 14.0527) knots 0 0 0 1 1 1
  spline S170 degree 2 poles (-16.9544, 14.0527) (-16.9544, 13.9958) (-16.9677, 13.9518) knots 0 0 0 1 1 1
  spline S171 degree 2 poles (-16.9677, 13.9518) (-16.981, 13.9078) (-17.0018, 13.879) knots 0 0 0 1 1 1
  spline S172 degree 2 poles (-17.0018, 13.879) (-17.0226, 13.8501) (-17.0474, 13.8336) knots 0 0 0 1 1 1
  spline S173 degree 2 poles (-17.0474, 13.8336) (-17.0721, 13.8171) (-17.1071, 13.8085) knots 0 0 0 1 1 1
  spline S174 degree 2 poles (-17.1071, 13.8085) (-17.142, 13.8) (-17.1874, 13.8) knots 0 0 0 1 1 1
  line L235 (-17.1874, 13.8) -> (-17.3678, 13.8)
  line L236 (-17.3016, 13.859) -> (-17.1949, 13.859)
  spline S175 degree 2 poles (-17.1949, 13.859) (-17.1454, 13.859) (-17.1173, 13.8682) knots 0 0 0 1 1 1
  spline S176 degree 2 poles (-17.1173, 13.8682) (-17.0891, 13.8774) (-17.0724, 13.8941) knots 0 0 0 1 1 1
  spline S177 degree 2 poles (-17.0724, 13.8941) (-17.0489, 13.9177) (-17.0358, 13.9574) knots 0 0 0 1 1 1
  spline S178 degree 2 poles (-17.0358, 13.9574) (-17.0226, 13.9971) (-17.0226, 14.0538) knots 0 0 0 1 1 1
  spline S179 degree 2 poles (-17.0226, 14.0538) (-17.0226, 14.1322) (-17.0484, 14.1743) knots 0 0 0 1 1 1
  spline S180 degree 2 poles (-17.0484, 14.1743) (-17.0741, 14.2164) (-17.111, 14.2308) knots 0 0 0 1 1 1
  spline S181 degree 2 poles (-17.111, 14.2308) (-17.1376, 14.241) (-17.1966, 14.241) knots 0 0 0 1 1 1
  line L237 (-17.1966, 14.241) -> (-17.3016, 14.241)
  line L238 (-17.3016, 14.241) -> (-17.3016, 13.859)
  spline S182 degree 2 poles (-16.8883, 14.0466) (-16.8883, 14.1353) (-16.87, 14.1893) knots 0 0 0 1 1 1
  spline S183 degree 2 poles (-16.87, 14.1893) (-16.8518, 14.2434) (-16.8158, 14.2727) knots 0 0 0 1 1 1
  spline S184 degree 2 poles (-16.8158, 14.2727) (-16.7798, 14.302) (-16.7252, 14.302) knots 0 0 0 1 1 1
  spline S185 degree 2 poles (-16.7252, 14.302) (-16.685, 14.302) (-16.6546, 14.2858) knots 0 0 0 1 1 1
  spline S186 degree 2 poles (-16.6546, 14.2858) (-16.6243, 14.2696) (-16.6045, 14.2391) knots 0 0 0 1 1 1
  spline S187 degree 2 poles (-16.6045, 14.2391) (-16.5847, 14.2086) (-16.5735, 14.1648) knots 0 0 0 1 1 1
  spline S188 degree 2 poles (-16.5735, 14.1648) (-16.5622, 14.1209) (-16.5622, 14.0466) knots 0 0 0 1 1 1
  spline S189 degree 2 poles (-16.5622, 14.0466) (-16.5622, 13.9586) (-16.5803, 13.9045) knots 0 0 0 1 1 1
  spline S190 degree 2 poles (-16.5803, 13.9045) (-16.5984, 13.8505) (-16.6343, 13.821) knots 0 0 0 1 1 1
  spline S191 degree 2 poles (-16.6343, 13.821) (-16.6703, 13.7915) (-16.7252, 13.7915) knots 0 0 0 1 1 1
  spline S192 degree 2 poles (-16.7252, 13.7915) (-16.7975, 13.7915) (-16.8388, 13.8433) knots 0 0 0 1 1 1
  spline S193 degree 2 poles (-16.8388, 13.8433) (-16.8883, 13.9057) (-16.8883, 14.0466) knots 0 0 0 1 1 1
  spline S194 degree 2 poles (-16.8252, 14.0466) (-16.8252, 13.9235) (-16.7963, 13.8827) knots 0 0 0 1 1 1
  spline S195 degree 2 poles (-16.7963, 13.8827) (-16.7675, 13.842) (-16.7252, 13.842) knots 0 0 0 1 1 1
  spline S196 degree 2 poles (-16.7252, 13.842) (-16.6829, 13.842) (-16.6541, 13.8829) knots 0 0 0 1 1 1
  spline S197 degree 2 poles (-16.6541, 13.8829) (-16.6253, 13.9238) (-16.6253, 14.0466) knots 0 0 0 1 1 1
  spline S198 degree 2 poles (-16.6253, 14.0466) (-16.6253, 14.1701) (-16.6541, 14.2106) knots 0 0 0 1 1 1
  spline S199 degree 2 poles (-16.6541, 14.2106) (-16.6829, 14.2512) (-16.7259, 14.2512) knots 0 0 0 1 1 1
  spline S200 degree 2 poles (-16.7259, 14.2512) (-16.7682, 14.2512) (-16.7934, 14.2154) knots 0 0 0 1 1 1
  spline S201 degree 2 poles (-16.7934, 14.2154) (-16.8252, 14.1697) (-16.8252, 14.0466) knots 0 0 0 1 1 1
  line L239 (-14.7637, 13.8) -> (-14.7637, 14.3)
  line L240 (-14.7637, 14.3) -> (-14.5915, 14.3)
  spline S202 degree 2 poles (-14.5915, 14.3) (-14.5332, 14.3) (-14.5025, 14.2928) knots 0 0 0 1 1 1
  spline S203 degree 2 poles (-14.5025, 14.2928) (-14.4595, 14.2829) (-14.4291, 14.257) knots 0 0 0 1 1 1
  spline S204 degree 2 poles (-14.4291, 14.257) (-14.3896, 14.2236) (-14.37, 14.1716) knots 0 0 0 1 1 1
  spline S205 degree 2 poles (-14.37, 14.1716) (-14.3504, 14.1196) (-14.3504, 14.0527) knots 0 0 0 1 1 1
  spline S206 degree 2 poles (-14.3504, 14.0527) (-14.3504, 13.9958) (-14.3637, 13.9518) knots 0 0 0 1 1 1
  spline S207 degree 2 poles (-14.3637, 13.9518) (-14.377, 13.9078) (-14.3978, 13.879) knots 0 0 0 1 1 1
  spline S208 degree 2 poles (-14.3978, 13.879) (-14.4186, 13.8501) (-14.4433, 13.8336) knots 0 0 0 1 1 1
  spline S209 degree 2 poles (-14.4433, 13.8336) (-14.468, 13.8171) (-14.503, 13.8085) knots 0 0 0 1 1 1
  spline S210 degree 2 poles (-14.503, 13.8085) (-14.5379, 13.8) (-14.5833, 13.8) knots 0 0 0 1 1 1
  line L241 (-14.5833, 13.8) -> (-14.7637, 13.8)
  line L242 (-14.6976, 13.859) -> (-14.5908, 13.859)
  spline S211 degree 2 poles (-14.5908, 13.859) (-14.5413, 13.859) (-14.5132, 13.8682) knots 0 0 0 1 1 1
  spline S212 degree 2 poles (-14.5132, 13.8682) (-14.4851, 13.8774) (-14.4684, 13.8941) knots 0 0 0 1 1 1
  spline S213 degree 2 poles (-14.4684, 13.8941) (-14.4448, 13.9177) (-14.4317, 13.9574) knots 0 0 0 1 1 1
  spline S214 degree 2 poles (-14.4317, 13.9574) (-14.4186, 13.9971) (-14.4186, 14.0538) knots 0 0 0 1 1 1
  spline S215 degree 2 poles (-14.4186, 14.0538) (-14.4186, 14.1322) (-14.4443, 14.1743) knots 0 0 0 1 1 1
  spline S216 degree 2 poles (-14.4443, 14.1743) (-14.4701, 14.2164) (-14.5069, 14.2308) knots 0 0 0 1 1 1
  spline S217 degree 2 poles (-14.5069, 14.2308) (-14.5335, 14.241) (-14.5925, 14.241) knots 0 0 0 1 1 1
  line L243 (-14.5925, 14.241) -> (-14.6976, 14.241)
  line L244 (-14.6976, 14.241) -> (-14.6976, 13.859)
  line L245 (-14.0529, 13.8) -> (-14.1143, 13.8)
  line L246 (-14.1143, 13.8) -> (-14.1143, 14.1912)
  spline S218 degree 2 poles (-14.1143, 14.1912) (-14.1365, 14.1701) (-14.1725, 14.1489) knots 0 0 0 1 1 1
  spline S219 degree 2 poles (-14.1725, 14.1489) (-14.2085, 14.1278) (-14.2371, 14.1172) knots 0 0 0 1 1 1
  line L247 (-14.2371, 14.1172) -> (-14.2371, 14.1765)
  spline S220 degree 2 poles (-14.2371, 14.1765) (-14.1856, 14.2008) (-14.1471, 14.2352) knots 0 0 0 1 1 1
  spline S221 degree 2 poles (-14.1471, 14.2352) (-14.1085, 14.2696) (-14.0925, 14.302) knots 0 0 0 1 1 1
  line L248 (-14.0925, 14.302) -> (-14.0529, 14.302)
  line L249 (-14.0529, 14.302) -> (-14.0529, 13.8)
  line L250 (-12.2528, 13.8) -> (-12.2528, 14.3)
  line L251 (-12.2528, 14.3) -> (-12.0805, 14.3)
  spline S222 degree 2 poles (-12.0805, 14.3) (-12.0222, 14.3) (-11.9915, 14.2928) knots 0 0 0 1 1 1
  spline S223 degree 2 poles (-11.9915, 14.2928) (-11.9485, 14.2829) (-11.9182, 14.257) knots 0 0 0 1 1 1
  spline S224 degree 2 poles (-11.9182, 14.257) (-11.8786, 14.2236) (-11.859, 14.1716) knots 0 0 0 1 1 1
  spline S225 degree 2 poles (-11.859, 14.1716) (-11.8394, 14.1196) (-11.8394, 14.0527) knots 0 0 0 1 1 1
  spline S226 degree 2 poles (-11.8394, 14.0527) (-11.8394, 13.9958) (-11.8527, 13.9518) knots 0 0 0 1 1 1
  spline S227 degree 2 poles (-11.8527, 13.9518) (-11.866, 13.9078) (-11.8868, 13.879) knots 0 0 0 1 1 1
  spline S228 degree 2 poles (-11.8868, 13.879) (-11.9076, 13.8501) (-11.9323, 13.8336) knots 0 0 0 1 1 1
  spline S229 degree 2 poles (-11.9323, 13.8336) (-11.9571, 13.8171) (-11.992, 13.8085) knots 0 0 0 1 1 1
  spline S230 degree 2 poles (-11.992, 13.8085) (-12.027, 13.8) (-12.0723, 13.8) knots 0 0 0 1 1 1
  line L252 (-12.0723, 13.8) -> (-12.2528, 13.8)
  line L253 (-12.1866, 13.859) -> (-12.0798, 13.859)
  spline S231 degree 2 poles (-12.0798, 13.859) (-12.0304, 13.859) (-12.0022, 13.8682) knots 0 0 0 1 1 1
  spline S232 degree 2 poles (-12.0022, 13.8682) (-11.9741, 13.8774) (-11.9574, 13.8941) knots 0 0 0 1 1 1
  spline S233 degree 2 poles (-11.9574, 13.8941) (-11.9339, 13.9177) (-11.9207, 13.9574) knots 0 0 0 1 1 1
  spline S234 degree 2 poles (-11.9207, 13.9574) (-11.9076, 13.9971) (-11.9076, 14.0538) knots 0 0 0 1 1 1
  spline S235 degree 2 poles (-11.9076, 14.0538) (-11.9076, 14.1322) (-11.9334, 14.1743) knots 0 0 0 1 1 1
  spline S236 degree 2 poles (-11.9334, 14.1743) (-11.9591, 14.2164) (-11.9959, 14.2308) knots 0 0 0 1 1 1
  spline S237 degree 2 poles (-11.9959, 14.2308) (-12.0225, 14.241) (-12.0815, 14.241) knots 0 0 0 1 1 1
  line L254 (-12.0815, 14.241) -> (-12.1866, 14.241)
  line L255 (-12.1866, 14.241) -> (-12.1866, 13.859)
  line L256 (-11.4506, 13.859) -> (-11.4506, 13.8)
  line L257 (-11.4506, 13.8) -> (-11.7811, 13.8)
  spline S238 degree 2 poles (-11.7811, 13.8) (-11.7817, 13.8222) (-11.7739, 13.8426) knots 0 0 0 1 1 1
  spline S239 degree 2 poles (-11.7739, 13.8426) (-11.7613, 13.8764) (-11.7335, 13.9091) knots 0 0 0 1 1 1
  spline S240 degree 2 poles (-11.7335, 13.9091) (-11.7057, 13.9419) (-11.6532, 13.9849) knots 0 0 0 1 1 1
  spline S241 degree 2 poles (-11.6532, 13.9849) (-11.5717, 14.0517) (-11.543, 14.0908) knots 0 0 0 1 1 1
  spline S242 degree 2 poles (-11.543, 14.0908) (-11.5144, 14.1298) (-11.5144, 14.1646) knots 0 0 0 1 1 1
  spline S243 degree 2 poles (-11.5144, 14.1646) (-11.5144, 14.2011) (-11.5404, 14.2262) knots 0 0 0 1 1 1
  spline S244 degree 2 poles (-11.5404, 14.2262) (-11.5665, 14.2512) (-11.6085, 14.2512) knots 0 0 0 1 1 1
  spline S245 degree 2 poles (-11.6085, 14.2512) (-11.6528, 14.2512) (-11.6794, 14.2246) knots 0 0 0 1 1 1
  spline S246 degree 2 poles (-11.6794, 14.2246) (-11.706, 14.198) (-11.7064, 14.151) knots 0 0 0 1 1 1
  line L258 (-11.7064, 14.151) -> (-11.7695, 14.1574)
  spline S247 degree 2 poles (-11.7695, 14.1574) (-11.763, 14.228) (-11.7207, 14.265) knots 0 0 0 1 1 1
  spline S248 degree 2 poles (-11.7207, 14.265) (-11.6784, 14.302) (-11.6071, 14.302) knots 0 0 0 1 1 1
  spline S249 degree 2 poles (-11.6071, 14.302) (-11.5352, 14.302) (-11.4932, 14.2621) knots 0 0 0 1 1 1
  spline S250 degree 2 poles (-11.4932, 14.2621) (-11.4513, 14.2222) (-11.4513, 14.1632) knots 0 0 0 1 1 1
  spline S251 degree 2 poles (-11.4513, 14.1632) (-11.4513, 14.1332) (-11.4635, 14.1042) knots 0 0 0 1 1 1
  spline S252 degree 2 poles (-11.4635, 14.1042) (-11.4758, 14.0752) (-11.5043, 14.0432) knots 0 0 0 1 1 1
  spline S253 degree 2 poles (-11.5043, 14.0432) (-11.5328, 14.0111) (-11.5989, 13.9552) knots 0 0 0 1 1 1
  spline S254 degree 2 poles (-11.5989, 13.9552) (-11.6542, 13.9088) (-11.6699, 13.8923) knots 0 0 0 1 1 1
  spline S255 degree 2 poles (-11.6699, 13.8923) (-11.6856, 13.8757) (-11.6958, 13.859) knots 0 0 0 1 1 1
  line L259 (-11.6958, 13.859) -> (-11.4506, 13.859)
  line L260 (-9.6986, 13.8) -> (-9.6986, 14.3)
  line L261 (-9.6986, 14.3) -> (-9.5264, 14.3)
  spline S256 degree 2 poles (-9.5264, 14.3) (-9.4681, 14.3) (-9.4374, 14.2928) knots 0 0 0 1 1 1
  spline S257 degree 2 poles (-9.4374, 14.2928) (-9.3944, 14.2829) (-9.3641, 14.257) knots 0 0 0 1 1 1
  spline S258 degree 2 poles (-9.3641, 14.257) (-9.3245, 14.2236) (-9.3049, 14.1716) knots 0 0 0 1 1 1
  spline S259 degree 2 poles (-9.3049, 14.1716) (-9.2853, 14.1196) (-9.2853, 14.0527) knots 0 0 0 1 1 1
  spline S260 degree 2 poles (-9.2853, 14.0527) (-9.2853, 13.9958) (-9.2986, 13.9518) knots 0 0 0 1 1 1
  spline S261 degree 2 poles (-9.2986, 13.9518) (-9.3119, 13.9078) (-9.3327, 13.879) knots 0 0 0 1 1 1
  spline S262 degree 2 poles (-9.3327, 13.879) (-9.3535, 13.8501) (-9.3782, 13.8336) knots 0 0 0 1 1 1
  spline S263 degree 2 poles (-9.3782, 13.8336) (-9.4029, 13.8171) (-9.4379, 13.8085) knots 0 0 0 1 1 1
  spline S264 degree 2 poles (-9.4379, 13.8085) (-9.4729, 13.8) (-9.5182, 13.8) knots 0 0 0 1 1 1
  line L262 (-9.5182, 13.8) -> (-9.6986, 13.8)
  line L263 (-9.6325, 13.859) -> (-9.5257, 13.859)
  spline S265 degree 2 poles (-9.5257, 13.859) (-9.4763, 13.859) (-9.4481, 13.8682) knots 0 0 0 1 1 1
  spline S266 degree 2 poles (-9.4481, 13.8682) (-9.42, 13.8774) (-9.4033, 13.8941) knots 0 0 0 1 1 1
  spline S267 degree 2 poles (-9.4033, 13.8941) (-9.3798, 13.9177) (-9.3666, 13.9574) knots 0 0 0 1 1 1
  spline S268 degree 2 poles (-9.3666, 13.9574) (-9.3535, 13.9971) (-9.3535, 14.0538) knots 0 0 0 1 1 1
  spline S269 degree 2 poles (-9.3535, 14.0538) (-9.3535, 14.1322) (-9.3792, 14.1743) knots 0 0 0 1 1 1
  spline S270 degree 2 poles (-9.3792, 14.1743) (-9.405, 14.2164) (-9.4418, 14.2308) knots 0 0 0 1 1 1
  spline S271 degree 2 poles (-9.4418, 14.2308) (-9.4684, 14.241) (-9.5274, 14.241) knots 0 0 0 1 1 1
  line L264 (-9.5274, 14.241) -> (-9.6325, 14.241)
  line L265 (-9.6325, 14.241) -> (-9.6325, 13.859)
  line L266 (-9.2188, 13.932) -> (-9.1574, 13.9402)
  spline S272 degree 2 poles (-9.1574, 13.9402) (-9.1468, 13.888) (-9.1214, 13.865) knots 0 0 0 1 1 1
  spline S273 degree 2 poles (-9.1214, 13.865) (-9.096, 13.842) (-9.0595, 13.842) knots 0 0 0 1 1 1
  spline S274 degree 2 poles (-9.0595, 13.842) (-9.0162, 13.842) (-8.9863, 13.872) knots 0 0 0 1 1 1
  spline S275 degree 2 poles (-8.9863, 13.872) (-8.9565, 13.902) (-8.9565, 13.9463) knots 0 0 0 1 1 1
  spline S276 degree 2 poles (-8.9565, 13.9463) (-8.9565, 13.9886) (-8.9841, 14.0161) knots 0 0 0 1 1 1
  spline S277 degree 2 poles (-8.9841, 14.0161) (-9.0117, 14.0435) (-9.0544, 14.0435) knots 0 0 0 1 1 1
  spline S278 degree 2 poles (-9.0544, 14.0435) (-9.0718, 14.0435) (-9.0977, 14.0367) knots 0 0 0 1 1 1
  line L267 (-9.0977, 14.0367) -> (-9.0909, 14.0906)
  spline S279 degree 2 poles (-9.0909, 14.0906) (-9.0847, 14.0899) (-9.081, 14.0899) knots 0 0 0 1 1 1
  spline S280 degree 2 poles (-9.081, 14.0899) (-9.0418, 14.0899) (-9.0104, 14.1104) knots 0 0 0 1 1 1
  spline S281 degree 2 poles (-9.0104, 14.1104) (-8.979, 14.1308) (-8.979, 14.1735) knots 0 0 0 1 1 1
  spline S282 degree 2 poles (-8.979, 14.1735) (-8.979, 14.2072) (-9.0019, 14.2294) knots 0 0 0 1 1 1
  spline S283 degree 2 poles (-9.0019, 14.2294) (-9.0247, 14.2516) (-9.0609, 14.2516) knots 0 0 0 1 1 1
  spline S284 degree 2 poles (-9.0609, 14.2516) (-9.0967, 14.2516) (-9.1205, 14.2291) knots 0 0 0 1 1 1
  spline S285 degree 2 poles (-9.1205, 14.2291) (-9.1444, 14.2065) (-9.1512, 14.1615) knots 0 0 0 1 1 1
  line L268 (-9.1512, 14.1615) -> (-9.2126, 14.1724)
  spline S286 degree 2 poles (-9.2126, 14.1724) (-9.2014, 14.2342) (-9.1615, 14.2681) knots 0 0 0 1 1 1
  spline S287 degree 2 poles (-9.1615, 14.2681) (-9.1216, 14.302) (-9.0622, 14.302) knots 0 0 0 1 1 1
  spline S288 degree 2 poles (-9.0622, 14.302) (-9.0213, 14.302) (-8.9868, 14.2845) knots 0 0 0 1 1 1
  spline S289 degree 2 poles (-8.9868, 14.2845) (-8.9524, 14.2669) (-8.9342, 14.2366) knots 0 0 0 1 1 1
  spline S290 degree 2 poles (-8.9342, 14.2366) (-8.9159, 14.2062) (-8.9159, 14.1721) knots 0 0 0 1 1 1
  spline S291 degree 2 poles (-8.9159, 14.1721) (-8.9159, 14.1397) (-8.9333, 14.1131) knots 0 0 0 1 1 1
  spline S292 degree 2 poles (-8.9333, 14.1131) (-8.9507, 14.0865) (-8.9848, 14.0708) knots 0 0 0 1 1 1
  spline S293 degree 2 poles (-8.9848, 14.0708) (-8.9405, 14.0606) (-8.9159, 14.0283) knots 0 0 0 1 1 1
  spline S294 degree 2 poles (-8.9159, 14.0283) (-8.8914, 13.9961) (-8.8914, 13.9477) knots 0 0 0 1 1 1
  spline S295 degree 2 poles (-8.8914, 13.9477) (-8.8914, 13.8822) (-8.9391, 13.8367) knots 0 0 0 1 1 1
  spline S296 degree 2 poles (-8.9391, 13.8367) (-8.9868, 13.7911) (-9.0598, 13.7911) knots 0 0 0 1 1 1
  spline S297 degree 2 poles (-9.0598, 13.7911) (-9.1257, 13.7911) (-9.1691, 13.8304) knots 0 0 0 1 1 1
  spline S298 degree 2 poles (-9.1691, 13.8304) (-9.2126, 13.8696) (-9.2188, 13.932) knots 0 0 0 1 1 1
  line L269 (-7.141, 13.8) -> (-7.141, 14.3)
  line L270 (-7.141, 14.3) -> (-6.9687, 14.3)
  spline S299 degree 2 poles (-6.9687, 14.3) (-6.9104, 14.3) (-6.8797, 14.2928) knots 0 0 0 1 1 1
  spline S300 degree 2 poles (-6.8797, 14.2928) (-6.8367, 14.2829) (-6.8064, 14.257) knots 0 0 0 1 1 1
  spline S301 degree 2 poles (-6.8064, 14.257) (-6.7668, 14.2236) (-6.7472, 14.1716) knots 0 0 0 1 1 1
  spline S302 degree 2 poles (-6.7472, 14.1716) (-6.7276, 14.1196) (-6.7276, 14.0527) knots 0 0 0 1 1 1
  spline S303 degree 2 poles (-6.7276, 14.0527) (-6.7276, 13.9958) (-6.7409, 13.9518) knots 0 0 0 1 1 1
  spline S304 degree 2 poles (-6.7409, 13.9518) (-6.7542, 13.9078) (-6.775, 13.879) knots 0 0 0 1 1 1
  spline S305 degree 2 poles (-6.775, 13.879) (-6.7958, 13.8501) (-6.8205, 13.8336) knots 0 0 0 1 1 1
  spline S306 degree 2 poles (-6.8205, 13.8336) (-6.8453, 13.8171) (-6.8802, 13.8085) knots 0 0 0 1 1 1
  spline S307 degree 2 poles (-6.8802, 13.8085) (-6.9152, 13.8) (-6.9605, 13.8) knots 0 0 0 1 1 1
  line L271 (-6.9605, 13.8) -> (-7.141, 13.8)
  line L272 (-7.0748, 13.859) -> (-6.968, 13.859)
  spline S308 degree 2 poles (-6.968, 13.859) (-6.9186, 13.859) (-6.8904, 13.8682) knots 0 0 0 1 1 1
  spline S309 degree 2 poles (-6.8904, 13.8682) (-6.8623, 13.8774) (-6.8456, 13.8941) knots 0 0 0 1 1 1
  spline S310 degree 2 poles (-6.8456, 13.8941) (-6.8221, 13.9177) (-6.8089, 13.9574) knots 0 0 0 1 1 1
  spline S311 degree 2 poles (-6.8089, 13.9574) (-6.7958, 13.9971) (-6.7958, 14.0538) knots 0 0 0 1 1 1
  spline S312 degree 2 poles (-6.7958, 14.0538) (-6.7958, 14.1322) (-6.8216, 14.1743) knots 0 0 0 1 1 1
  spline S313 degree 2 poles (-6.8216, 14.1743) (-6.8473, 14.2164) (-6.8841, 14.2308) knots 0 0 0 1 1 1
  spline S314 degree 2 poles (-6.8841, 14.2308) (-6.9107, 14.241) (-6.9697, 14.241) knots 0 0 0 1 1 1
  line L273 (-6.9697, 14.241) -> (-7.0748, 14.241)